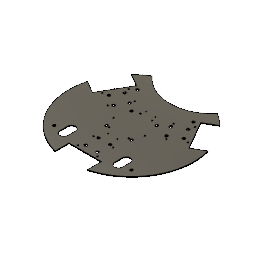
Plate_Mid (Autodesk Fusion 360 design; units mm, degrees)
Autodesk Fusion 360 part; units mm, degrees
sketch "Esboço1" plane through (0, 0, 0) normal (0, 0, 1) x (1, 0, 0)
  circle A0 centre (0, 0) radius 240
  line L0 (48, -48) -> (-48, -48)
  line L1 (-48, -48) -> (-48, 48)
  line L2 (-48, 48) -> (48, 48)
  line L3 (48, 48) -> (48, -48)
  line L4 (48, -48) -> (-48, 48) construction
  line L5 (-48, -48) -> (48, 48) construction
  circle A1 centre (-48, 48) radius 5
  circle A2 centre (-48, -48) radius 5
  circle A3 centre (48, 48) radius 5
  circle A4 centre (48, -48) radius 5
  line L6 (105, -110) -> (105, -170)
  line L7 (90, -125) -> (90, -155)
  line L8 (120, -125) -> (120, -155)
  arc A5 (120, -125) -> (90, -125) centre (105, -125) ccw
  arc A6 (90, -155) -> (120, -155) centre (105, -155) ccw
  circle A7 centre (148, -148) radius 5
  line L9 (-125, 204.878) -> (125, 204.878)
  circle A8 centre (0, 311.043) radius 164
  circle A9 centre (107.5, 130.5) radius 5
  line L10 (-40, 115) -> (40, 115)
  line L11 (-40, 115) -> (-40, 151.9958)
  line L12 (40, 115) -> (40, 151.9958)
  line L13 (0, 1.75) -> (0, 22.5)
  line L14 (-120, -125) -> (-120, -155)
  arc A10 (-90, -125) -> (-120, -125) centre (-105, -125) ccw
  line L15 (-90, -125) -> (-90, -155)
  arc A11 (-120, -155) -> (-90, -155) centre (-105, -155) ccw
  circle A12 centre (-148, -148) radius 5
  circle A13 centre (-107.5, 130.5) radius 5
  line L16 (-61.5, -178) -> (61.5, -178)
  line L17 (61.5, -178) -> (61.5, -240)
  line L18 (61.5, -240) -> (-61.5, -240)
  line L19 (-61.5, -240) -> (-61.5, -178)
  line L20 (0, -178) -> (0, -168)
  line L21 (-37.5, -168) -> (37.5, -168)
  circle A14 centre (-37.5, -168) radius 2.5
  circle A15 centre (37.5, -168) radius 2.5
  circle A16 centre (37.5, -108) radius 2.5
  circle A17 centre (37.5, -48) radius 2.5
  circle A18 centre (-37.5, -108) radius 2.5
  circle A19 centre (-37.5, -48) radius 2.5
  circle A20 centre (126.7423, 116.476) radius 2.5
  line L22 (238.5961, 66.7394) -> (184.9025, 35.7394)
  line L23 (184.9025, 35.7394) -> (123.4025, 142.2606)
  line L24 (123.4025, 142.2606) -> (177.0961, 173.2606)
  circle A21 centre (74.7807, 86.476) radius 2.5
  circle A22 centre (164.2423, 51.524) radius 2.5
  circle A23 centre (112.2807, 21.524) radius 2.5
  circle A24 centre (60.3192, -8.476) radius 2.5
  circle A25 centre (22.8192, 56.476) radius 2.5
  circle A26 centre (-164.2423, 51.524) radius 2.5
  line L25 (-177.0961, 173.2606) -> (-123.4025, 142.2606)
  line L26 (-123.4025, 142.2606) -> (-184.9025, 35.7394)
  line L27 (-184.9025, 35.7394) -> (-238.5961, 66.7394)
  circle A27 centre (-112.2807, 21.524) radius 2.5
  circle A28 centre (-126.7423, 116.476) radius 2.5
  circle A29 centre (-74.7807, 86.476) radius 2.5
  circle A30 centre (-22.8192, 56.476) radius 2.5
  circle A31 centre (-60.3192, -8.476) radius 2.5
  line L28 (0, -178) -> (0, -153)
  line L29 (-22.5, -153) -> (22.5, -153)
  circle A32 centre (-22.5, -153) radius 5
  circle A33 centre (22.5, -153) radius 5
  circle A34 centre (-22.5, -104) radius 5
  circle A35 centre (22.5, -104) radius 5
  circle A36 centre (143.7519, 57.0144) radius 5
  circle A37 centre (101.3166, 32.5144) radius 5
  circle A38 centre (78.8166, 71.4856) radius 5
  circle A39 centre (121.2519, 95.9856) radius 5
  circle A40 centre (-121.2519, 95.9856) radius 5
  circle A41 centre (-78.8166, 71.4856) radius 5
  circle A42 centre (-101.3166, 32.5144) radius 5
  circle A43 centre (-143.7519, 57.0144) radius 5
  line L30 (-17.902, -72) -> (18.098, -72)
  circle A44 centre (-17.902, -72) radius 1.75
  circle A45 centre (18.098, -72) radius 1.75
  line L31 (0, 311.043) -> (0, 115)
  circle A46 centre (-17.902, 74) radius 1.75
  circle A47 centre (18.098, 74) radius 1.75
  point P0 (105, -110)
  point P1 (0, 115)
  point P2 (0, -240)
  point P3 (-61.5, -231.9865)
  point P4 (-170.1562, 169.2538)
  point P5 (170.1562, 169.2538)
  point P6 (0.098, -72)
  dimension "d1" = 480
  dimension "d2" = 96
  dimension "d3" = 96
  dimension "d4" = 10
  dimension "d5" = 10
  dimension "d6" = 10
  dimension "d7" = 10
  dimension "d8" = 110
  dimension "d9" = 105
  dimension "d10" = 30
  dimension "d11" = 60
  dimension "d12" = 30
  dimension "d13" = 10
  dimension "d14" = 148
  dimension "d15" = 148
  dimension "d16" = 250
  dimension "d17" = 328
  dimension "d18" = 10
  dimension "d19" = 130.5
  dimension "d20" = 107.5
  dimension "d21" = 115
  dimension "d22" = 80
  dimension "d25" = 123
  dimension "d26" = 62
  dimension "d27" = 10
  dimension "d28" = 75
  dimension "d29" = 5
  dimension "d30" = 5
  dimension "d33" = 1
  dimension "d34" = 60
  dimension "d36" = 360
  dimension "d37" = 25
  dimension "d38" = 45
  dimension "d39" = 10
  dimension "d40" = 10
  dimension "d43" = 0
  dimension "d44" = 49
  dimension "d45" = 36
  dimension "d46" = 3.5
  dimension "d47" = 3.5
  dimension "d51" = 0
  dimension "d52" = 146
  dimension "d53" = 32
  constraint coincident A0.centre origin
  constraint horizontal L0
  constraint perpendicular L0 L1
  constraint parallel L0 L2
  constraint parallel L1 L3
  constraint coincident L4 A0.centre
  constraint coincident L5 A0.centre
  constraint coincident L1.end L2.start
  constraint coincident L0.end L1.start
  constraint coincident L2.end L3.start
  constraint coincident L0.start L3.end
  constraint coincident P0 A5
  constraint coincident P0 L6.start
  constraint vertical L6
  constraint coincident A5.centre L6
  constraint coincident L6.end A6
  constraint tangent L7 A6
  constraint parallel L6 L7
  constraint tangent L8 A6
  constraint parallel L6 L8
  constraint horizontal L9
  constraint coincident A0 L9.start
  constraint coincident A0 L9.end
  constraint coincident L9.start A8
  constraint coincident L9.end A8
  constraint horizontal L10
  constraint midpoint P1 L10
  constraint coincident A8 L11.end
  constraint perpendicular L10 L11
  constraint coincident A8 L12.end
  constraint perpendicular L10 L12
  constraint symmetric L7.start L13 A10.start
  constraint symmetric L7.end L13 L15.end
  constraint symmetric L8.start L13 L14.start
  constraint symmetric L8.end L13 L14.end
  constraint symmetric A5 L13 A10
  constraint symmetric A6 L13 A11
  constraint symmetric A7 L13 A12
  constraint symmetric A9 L13 A13
  constraint horizontal L16
  constraint vertical L17
  constraint horizontal L18
  constraint vertical L19
  constraint midpoint L18 P2
  constraint tangent A0 L18
  constraint coincident A0 P2
  constraint midpoint L16 L20.start
  constraint perpendicular L16 L20
  constraint horizontal L21
  constraint midpoint L20.end L21
  constraint coincident L21.start A14.centre
  constraint coincident L21.end A15.centre
  constraint coincident A0 P3
  constraint coincident L19 P3
  constraint coincident L25 P4
  constraint coincident A0 P4
  constraint coincident L24 P5
  constraint coincident A0 P5
  constraint perpendicular L21 L28
  constraint horizontal L29
  constraint midpoint L28.end L29
  constraint coincident L29.start A32.centre
  constraint coincident L29.end A33.centre
  constraint horizontal L30
  constraint coincident L30.start A44.centre
  constraint coincident L30.end A45.centre
  constraint coincident A8.centre L31.start
  constraint coincident P1 L31.end
  constraint vertical L31
  constraint midpoint L30 P6
  measures "d1" diameter of A0
  measures "d2" distance of L1.end L2.end
  measures "d3" distance of L0.end L1.end
  measures "d4" diameter of A1
  measures "d5" diameter of A2
  measures "d6" diameter of A3
  measures "d7" diameter of A4
  measures "d8" vertical distance of A0.centre P0
  measures "d9" horizontal distance of A0.centre P0
  measures "d10" diameter of A5
  measures "d11" distance of P0 L6.end
  measures "d12" diameter of A6
  measures "d13" diameter of A7
  measures "d14" vertical distance of A0.centre A7.centre
  measures "d15" horizontal distance of A0.centre A7.centre
  measures "d16" distance of L9.start L9.end
  measures "d17" diameter of A8
  measures "d18" diameter of A9
  measures "d19" vertical distance of A0.centre A9.centre
  measures "d20" horizontal distance of A0.centre A9.centre
  measures "d21" distance of A0.centre L31.end
  measures "d22" distance of L10.start L10.end
  measures "d25" distance of L16.start L16.end
  measures "d26" distance of L16.start L18.end
  measures "d27" distance of L20.start L20.end
  measures "d28" distance of L21.start L21.end
  measures "d29" diameter of A14
  measures "d30" diameter of A15
  measures "d37" distance of L20.start L28.end
  measures "d38" distance of L29.start L29.end
  measures "d39" diameter of A32
  measures "d40" diameter of A33 A3
  measures "d45" distance of L30.start L30.end
  measures "d46" diameter of A44
  measures "d47" diameter of A45
  measures "d53" vertical distance of A34.centre P6
extrude "Extrusão1" add sketch "Esboço1" along normal blind 3 contours A0 A8 L10 L11 L12 L16 L17 L19 L22 L23 L24 L25 L26 L27 | A8 L10 L12 L31 | A8 L10 L11 L31 | L0 L1 L2 L3 A1 A2 A3 A4 A17 A19
sketch "Esboço2" plane through (0, -178, 0) normal (0, -1, 0) x (1, 0, 0)
  line L0 (-61.5, 0) -> (61.5, 0)
  line L1 (61.5, 0) -> (61.5, 3)
  line L2 (61.5, 3) -> (-61.5, 3)
  line L3 (-61.5, 3) -> (-61.5, 0)
  line L4 (-61.5, 3) -> (61.5, 3)
  line L5 (61.5, 3) -> (61.5, 0)
  line L6 (61.5, 0) -> (-61.5, 0)
  line L7 (-61.5, 0) -> (-61.5, 3)
  line L8 (0, 3) -> (0, 0)
  line L9 (-61.5, 1.5) -> (61.5, 1.5)
  circle A0 centre (0, 1.5) radius 0.75
  dimension "d54" = 1.5
  constraint horizontal L4
  constraint vertical L5
  constraint horizontal L6
  constraint vertical L7
  constraint coincident L0.end L1.start
  constraint coincident L2.end L3.start
  constraint midpoint L2 L8.start
  constraint coincident L8.end origin
  constraint midpoint L3 L9.start
  constraint midpoint L1 L9.end
  constraint midpoint L9 A0.centre
  measures "d54" diameter of A0
sketch "Esboço3" plane through (154.1525, 89, 0) normal (0.866025, 0.5, 0) x (-0.5, 0.866025, 0)
  line L0 (-61.5, 0) -> (61.5, 0)
  line L1 (61.5, 0) -> (61.5, 3)
  line L2 (61.5, 3) -> (-61.5, 3)
  line L3 (-61.5, 3) -> (-61.5, 0)
  line L4 (-61.5, 3) -> (61.5, 3)
  line L5 (61.5, 3) -> (61.5, 0)
  line L6 (61.5, 0) -> (-61.5, 0)
  line L7 (-61.5, 0) -> (-61.5, 3)
  line L8 (-61.5, 1.5) -> (61.5, 1.5)
  line L9 (0, 3) -> (0, 0)
  circle A0 centre (0, 1.5) radius 0.75
  dimension "d55" = 1.5
  constraint horizontal L4
  constraint vertical L5
  constraint horizontal L6
  constraint vertical L7
  constraint coincident L0.end L1.start
  constraint coincident L2.end L3.start
  constraint midpoint L3 L8.start
  constraint midpoint L2 L9.start
  constraint coincident L9.end origin
  constraint midpoint L8 A0.centre
  constraint midpoint L1 L8.end
  measures "d55" diameter of A0
sketch "Esboço4" plane through (-154.1525, 89, 0) normal (-0.866025, 0.5, 0) x (-0.5, -0.866025, 0)
  line L0 (-61.5, 0) -> (61.5, 0)
  line L1 (61.5, 0) -> (61.5, 3)
  line L2 (61.5, 3) -> (-61.5, 3)
  line L3 (-61.5, 3) -> (-61.5, 0)
  line L4 (-61.5, 3) -> (61.5, 3)
  line L5 (61.5, 3) -> (61.5, 0)
  line L6 (61.5, 0) -> (-61.5, 0)
  line L7 (-61.5, 0) -> (-61.5, 3)
  line L8 (0, 3) -> (0, 0)
  line L9 (-61.5, 1.5) -> (61.5, 1.5)
  circle A0 centre (0, 1.5) radius 0.75
  dimension "d56" = 1.5
  constraint horizontal L4
  constraint vertical L5
  constraint horizontal L6
  constraint vertical L7
  constraint coincident L0.end L1.start
  constraint coincident L2.end L3.start
  constraint midpoint L2 L8.start
  constraint coincident L8.end origin
  constraint midpoint L3 L9.start
  constraint midpoint L1 L9.end
  constraint midpoint L9 A0.centre
  measures "d56" diameter of A0
extrude "Extrusão2" add sketch "Esboço4" along normal blind 5 contours L8 L9 A0 | L8 L9 A0 | L8 L9 A0 | L8 L9 A0
extrude "Extrusão3" add sketch "Esboço2" along normal blind 5 contours L8 L9 A0 | L8 L9 A0 | L8 L9 A0 | L8 L9 A0
extrude "Extrusão4" add sketch "Esboço3" along normal blind 5 contours L8 L9 A0 | L8 L9 A0 | L8 L9 A0 | L8 L9 A0
equation "d12 = d10"
equation "d17 = ( 164 * 2 ) * 1 mm"
